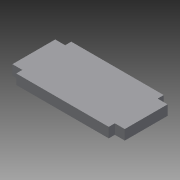
# Autodesk Inventor part: arm-servo
Saved by Autodesk Inventor 2013 (Build 170138000, 138)
## iProperties
Created: 2012-09-08
Part Number: arm-servo
Material: Generic
Document SubType Name: Modeling
Designer: frankenteddy
Density: 1 g/cm^3
Author: frankenteddy
Autodesk Inventor part; units mm, degrees
ref_plane "YZ Plane" through (0, 0, 0) normal (1, 0, 0) x (0, 1, 0)
ref_plane "XZ Plane" through (0, 0, 0) normal (0, 1, 0) x (-1, 0, 0)
ref_plane "XY Plane" through (0, 0, 0) normal (0, 0, 1) x (1, 0, 0)
sketch "Block1" plane through (0, 0, 0) normal (0, 0, 1) x (1, 0, 0)
  circle A0 centre (74.029, 24.2723) radius 1
  line L0 (49.279, 30.4723) -> (71.779, 30.4723)
  line L1 (71.779, 30.4723) -> (71.779, 18.0723)
  line L2 (71.779, 18.0723) -> (49.279, 18.0723)
  line L3 (49.279, 18.0723) -> (49.279, 30.4723)
  line L4 (49.279, 30.4723) -> (44.779, 30.4723)
  line L5 (44.779, 30.4723) -> (44.779, 18.0723)
  line L6 (44.779, 18.0723) -> (49.279, 18.0723)
  line L7 (49.279, 18.0723) -> (49.279, 30.4723)
  line L8 (71.779, 30.4723) -> (76.279, 30.4723)
  line L9 (76.279, 30.4723) -> (76.279, 18.0723)
  line L10 (76.279, 18.0723) -> (71.779, 18.0723)
  line L11 (71.779, 18.0723) -> (71.779, 30.4723)
  line L12 (44.779, 24.2723) -> (76.279, 24.2723) construction
  line L13 (47.029, 30.4723) -> (47.029, 18.0723) construction
  circle A1 centre (47.029, 24.2723) radius 1
  line L14 (74.029, 30.4723) -> (74.029, 18.0723) construction
  point P0 (60.979, 24.0984)
  dimension "d7" = 22.5
  dimension "d8" = 12.4
  dimension "d9" = 4.5
  dimension "d10" = 4.5
  dimension "d11" = 2
  dimension "d12" = 2
  measures "d7" distance of L1.end L2.end
  measures "d8" distance of L0.end L1.end
  measures "d9" distance of L6.end L5.end
  measures "d10" distance of L9.end L10.end
  measures "d11" diameter of A0
  measures "d12" diameter of A1
sketch "Sketch1" plane through (0, 0, 0) normal (0, 0, 1) x (1, 0, 0)
  line L0 (-92.7646, -8.503) -> (-89.7646, -8.503)
  line L1 (-89.7646, -8.503) -> (-89.7646, -11.753)
  line L2 (-89.7646, -11.753) -> (-92.7646, -11.753)
  line L3 (-92.7646, -11.753) -> (-92.7646, -8.503)
  line L4 (-92.7646, -21.6527) -> (-89.7646, -21.6527)
  line L5 (-89.7646, -21.6527) -> (-89.7646, -21.7527)
  line L6 (-89.7646, -21.7527) -> (-92.7646, -21.7527)
  line L7 (-92.7646, -21.7527) -> (-92.7646, -21.6527)
  line L8 (-37.803, 27.4868) -> (-7.553, 27.4868)
  line L9 (-7.553, 27.4868) -> (-7.553, 9.4868)
  line L10 (-7.553, 9.4868) -> (-37.803, 9.4868)
  line L11 (-37.803, 9.4868) -> (-37.803, 27.4868)
  line L12 (-41.053, 25.4868) -> (-37.803, 25.4868)
  line L13 (-37.803, 25.4868) -> (-37.803, 11.4868)
  line L14 (-37.803, 11.4868) -> (-41.053, 11.4868)
  line L15 (-41.053, 11.4868) -> (-41.053, 25.4868)
  line L16 (-37.803, 18.4868) -> (-7.553, 18.4868) construction
  line L17 (-22.678, 27.4868) -> (-22.678, 9.4868) construction
  line L18 (-41.053, 18.4868) -> (-37.803, 18.4868) construction
  line L19 (-4.303, 25.4868) -> (-7.553, 25.4868)
  line L20 (-7.553, 25.4868) -> (-7.553, 11.4868)
  line L21 (-7.553, 11.4868) -> (-4.303, 11.4868)
  line L22 (-4.303, 11.4868) -> (-4.303, 25.4868)
  line L23 (-4.303, 18.4868) -> (-7.553, 18.4868) construction
  point P0 (0, 0)
  point P1 (-7.553, 18.4868)
  dimension "d0" = 3
  dimension "mat" = 3.25
  dimension "d2" = 3
  dimension "d3" = 0.1
  dimension "d38" = 30.25
  dimension "d39" = 18
  dimension "d40" = 3.25
  dimension "d41" = 14
  constraints: 48 end point, 8 parallel, 7 symmetric about line, 6 midpoint, 4 horizontal, 4 perpendicular, 2 collinear
  measures "d0" distance of L1.end L3.start
  measures "mat" distance of L1.start L1.end
  measures "d2" distance of L5.end L7.start
  measures "d3" distance of L5.start L5.end
  measures "d38" distance of L9.end L10.end
  measures "d39" distance of L8.end L9.end
  measures "d40" distance of L13.end L14.end
  measures "d41" distance of L12.end L13.end
extrude "Extrusion5" add sketch "Sketch1" along normal blind 3.25 contours L8 L9 L10 L11 | L11 L14 L15 L12 | L19 L22 L21 L9
equation "\"d40\" = mat"
equation "\"d42\" = mat"
body "Solid5"
